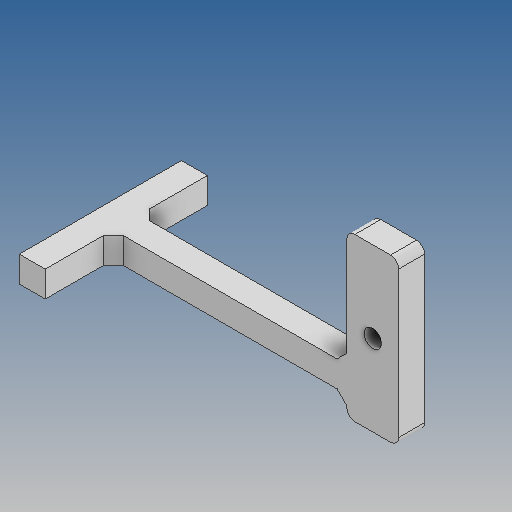
# Autodesk Inventor part: Gripper neu
Saved by Autodesk Inventor 2026.2 (Build 302298000, 298)
## iProperties
Created: 2025-12-08
Part Number: Gripper neu
Material: Generisch
Document SubType Name: Modeling
Designer: Schally
Density: 1 g/cm^3
Appearance: Vorgabe
Author: Schally
Autodesk Inventor part; units mm, degrees
ref_plane "YZ Plane" through (0, 0, 0) normal (1, 0, 0) x (0, 1, 0)
ref_plane "XZ Plane" through (0, 0, 0) normal (0, 1, 0) x (-1, 0, 0)
ref_plane "XY Plane" through (0, 0, 0) normal (0, 0, 1) x (1, 0, 0)
sketch "Skizze2" plane through (0, 0, 0) normal (0, 0, 1) x (1, 0, 0)
  line L0 (-19.9249, 0) -> (3.9249, 0) projected
  line L1 (0, -18.1036) -> (0, 108.6213) projected
  circle A0 centre (-8, 65) radius 2.7
  line L2 (0, 0) -> (0, 87.5)
  arc A1 (0, 87.5) -> (-2.5, 90) centre (-2.5, 87.5) ccw
  line L3 (-13.5, 90) -> (-2.5, 90)
  arc A2 (-13.5, 90) -> (-16, 87.5) centre (-13.5, 87.5) ccw
  line L4 (0, 42.5) -> (0, 87.5)
  line L5 (-16, 40) -> (-16, 87.5)
  line L6 (0, 40) -> (-16, 40)
  point P0 (-8, 90)
  dimension "d4" = 2.5
  dimension "d5" = 2.5
  dimension "d6" = 5.4
  dimension "d8" = 25
  dimension "d17" = 2.5
  dimension "d18" = 2.5
  dimension "d19" = 2.5
  dimension "d144" = 25
  constraints: 10 end point, 5 point on circle, 3 centre point, 3 point on line, 2 vertical, 1 midpoint, 1 parallel, 1 tangent
  measures "d4" radius of A1
  measures "d5" radius of A2
  measures "d6" diameter of A0
  measures "d8" distance from line of L3 A0.centre
  measures "d17" distance from line of A2.centre L3
  measures "d18" distance from line of A1.centre L3
  measures "d19" distance from line of A1.centre L1
  measures "d144" distance of point (-8, 90) A0.centre
extrude "Extrusion1" add sketch "Skizze2" along normal mid plane 8
sketch "Skizze7" plane through (0, 0, -4) normal (0, 0, -1) x (-1, 0, 0)
  arc A0 (16, 87.5) -> (13.5, 90) centre (13.5, 87.5) ccw projected
  line L0 (13.5, 90) -> (2.5, 90) projected
  arc A1 (2.5, 90) -> (0, 87.5) centre (2.5, 87.5) ccw projected
  line L1 (0, 87.5) -> (0, 40) projected
  circle A2 centre (8, 65) radius 2.7 projected
  circle A3 centre (8, 65) radius 6.5
  line L2 (8, 85) -> (8, 45)
  line L3 (13, 82.2483) -> (13, 48.2483)
  line L4 (3, 48.3648) -> (3, 82.3648)
  line L5 (16, 40) -> (16, 87.5) projected
  line L6 (0, 40) -> (16, 40) projected
  circle A4 centre (8, 82) radius 3
  circle A5 centre (8, 48) radius 3
  line L7 (-2, 82) -> (18, 82)
  line L8 (-2, 48) -> (18, 48)
  line L9 (5, 48) -> (3, 60.8467)
  line L10 (11, 48) -> (13, 60.8467)
  line L11 (3, 69.1533) -> (5, 82)
  line L12 (13, 69.1533) -> (11, 82)
  point P0 (0, 0)
  point P1 (8, 65)
  dimension "d133" = 13
  dimension "d136" = 20
  dimension "d137" = 20
  dimension "d194" = 6
  dimension "d195" = 6
  dimension "d196" = 3
  dimension "d197" = 3
  dimension "d198" = 10
  dimension "d199" = 20
  dimension "d200" = 20
  constraints: 18 end point, 10 point on line, 8 point on circle, 3 centre point, 3 midpoint, 2 horizontal, 2 vertical alignment, 1 coincident, 1 vertical, 1 other
  measures "d133" diameter of A3
  measures "d136" distance of A2.centre L2.start
  measures "d137" distance of L2.end A2.centre
  measures "d194" diameter of A4
  measures "d195" diameter of A5
  measures "d196" distance of L2.end A5.centre
  measures "d197" distance of A4.centre L2.start
  measures "d198" distance between parallel lines of L3 L4
  measures "d199" distance of L7.start L7.end
  measures "d200" distance of L8.start L8.end
extrude "Extrusion5" cut sketch "Skizze7" against normal blind 4 contours L8 L2 A5 | A5 L2 L8 | A5 L2 A3 L10 | L3 A3 L2 A2 | A3 L3 | A3 L2 A4 L12 | L7 L2 A4 | A4 L2 L7 | A5 L8 L2 | A5 L9 A3 L2 | L2 L8 A5 | L2 A2 A3 L4 | A3 L11 A4 L2 | L2 L7 A4 | A4 L7 L2 | L4 A3
fillet "Rundung2" radius 2.5 2 edges at (0, 40, 0) (-16, 40, 0)
sketch "Skizze12" plane through (-16, 40, 4) normal (-1, 0, 0) x (0, 0, 1)
  line L0 (0, 47.5) -> (0, 0) projected
  line L1 (-8, 0) -> (-8, 47.5) projected
  line L2 (0, 47.5) -> (0, 2.5) projected
  line L3 (-8, 47.5) -> (0, 47.5) projected
  line L4 (-8, 2.5) -> (-8, 47.5) projected
  line L5 (0, 6) -> (-8, 6)
  line L6 (-8, 6) -> (-8, 14)
  line L7 (-8, 14) -> (0, 14)
  line L8 (0, 14) -> (0, 6)
  line L9 (0, 2.5) -> (-8, 2.5) projected
  point P0 (-4, -40)
  point P1 (0, 8)
  point P2 (-4, 20.6699)
  point P3 (0, 14)
  dimension "d184" = 8
  constraints: 8 end point, 3 point on line, 2 parallel, 1 horizontal, 1 perpendicular
  measures "d184" distance of L5.end L6.end
extrude "Extrusion10" add sketch "Skizze12" along normal blind 80 contours L0 L5 L1 L7
sketch "Skizze17" plane through (-16, 54, 4) normal (0, 1, 0) x (1, 0, 0)
  line L0 (-80, 0) -> (-80, 8) projected
  line L1 (-72, 29) -> (-80, 29)
  line L2 (-72, -21) -> (-80, -21)
  line L3 (-80, 29) -> (-80, -21)
  line L4 (-72, 29) -> (-72, -21)
  line L5 (0, 8) -> (0, 0) projected
  line L6 (0, 8) -> (-80, 8) projected
  line L7 (-80, 0) -> (-80, 8) projected
  line L8 (0, 0) -> (-80, 0) projected
  line L9 (-80, 4) -> (0, 4)
  point P0 (16, 4)
  point P1 (-80, 8)
  dimension "d187" = 50
  dimension "d188" = 8
  constraints: 10 end point, 3 midpoint, 2 horizontal, 1 parallel, 1 vertical, 1 vertical alignment, 1 other
  measures "d187" distance of L1.end L2.end
  measures "d188" distance between parallel lines of L3 L4
extrude "Extrusion15" add sketch "Skizze17" against normal blind 8 contours L8 L4 L2 L3 | L0 L9 L4 L8 | L0 L6 L4 L9 | L3 L1 L4 L6
chamfer "Fasen10" distance 3 angle 45 4 edges at (-16, 46, 0) (-16, 54, 0) (-88, 50, -4) (-88, 50, 4)
